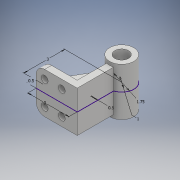
# Autodesk Inventor part: 7d
Saved by Autodesk Inventor 2018 (Build 220112000, 112)
## iProperties
Created: 2018-10-23
Part Number: 7d
Material: Generic
Document SubType Name: Modeling
Designer: Jerry
Density: 1 g/cm^3
Appearance: Default
Author: Jerry
Autodesk Inventor part; units mm, degrees
ref_plane "YZ Plane" through (0, 0, 0) normal (1, 0, 0) x (0, 1, 0)
ref_plane "XZ Plane" through (0, 0, 0) normal (0, 1, 0) x (-1, 0, 0)
ref_plane "XY Plane" through (0, 0, 0) normal (0, 0, 1) x (1, 0, 0)
sketch "Sketch1" plane through (0, 0, 0) normal (0, 0, 1) x (1, 0, 0)
  line L0 (0, 0) -> (0, 0.5)
  line L1 (0, 0.5) -> (2.5, 0.5)
  line L2 (2.5, 0.5) -> (2.5, 2.6615)
  line L3 (0, 0) -> (3, 0)
  line L4 (3, 0) -> (3, 2.6615)
  circle A0 centre (2.75, 3.5) radius 0.5
  circle A1 centre (2.75, 3.5) radius 0.875
  line L5 (0, 0.5) -> (1.993, 3.9388)
  dimension "d0" = 0.5
  dimension "d1" = 0.5
  dimension "d2" = 3
  dimension "d3" = 1
  dimension "d4" = 1.75
  dimension "d20" = 3
  constraints: 12 end point, 3 perpendicular, 3 point on circle, 2 centre point, 1 coincident, 1 horizontal, 1 horizontal alignment, 1 tangent, 1 vertical
  measures "d0" distance between parallel lines of L3 L1
  measures "d1" distance between parallel lines of L4 L2
  measures "d2" distance from line of L1 A0.centre
  measures "d3" diameter of A0
  measures "d4" diameter of A1
  measures "d20" distance from line of L0.start L4
sketch "Sketch2" plane through (0, 0, 0) normal (0, 1, 0) x (-1, 0, 0)
  line L0 (0.7553, 0) -> (-3.6259, 0) projected
  line L1 (0, 0) -> (0, -0.875)
  arc A0 (-0.625, -1.5) -> (0, -0.875) centre (-0.625, -0.875) ccw
  line L2 (-0.625, -1.5) -> (-3, -1.5)
  line L3 (-3, -1.5) -> (-3, 1.5)
  line L4 (-3, 1.5) -> (-0.625, 1.5)
  arc A1 (0, 0.875) -> (-0.625, 1.5) centre (-0.625, 0.875) ccw
  line L5 (0, 0.875) -> (0, 0)
  line L6 (0, -0.25) -> (-2.5, -0.25)
  line L7 (-2.5, -0.25) -> (-2.5, -1.5)
  line L8 (0, 0.25) -> (-2.5, 0.25)
  line L9 (-2.5, 0.25) -> (-2.5, 1.5)
  circle A2 centre (-0.625, -0.875) radius 0.25
  circle A3 centre (-1.875, -0.875) radius 0.25
  circle A4 centre (-0.625, 0.875) radius 0.25
  circle A5 centre (-1.875, 0.875) radius 0.25
  point P0 (-0.625, -0.875)
  point P1 (-1.875, -0.875)
  point P2 (-1.875, 0.875)
  point P3 (-0.625, 0.875)
  dimension "d5" = 1.75
  dimension "d6" = 1.25
  dimension "d7" = 0.625
  dimension "d8" = 1.25
  dimension "d9" = 2.5
  dimension "d10" = 3
  dimension "d11" = 0.5
  dimension "d14" = 1.25
  dimension "d17" = 1.75
  dimension "d21" = 3
  constraints: 18 end point, 7 perpendicular, 7 point on line, 6 centre point, 4 point on circle, 4 tangent, 2 coincident, 2 horizontal alignment, 2 vertical, 2 vertical alignment, 1 horizontal, 1 parallel, 1 symmetric about line, 10 other
  measures "d5" distance of point (-0.625, 0.875) point (-0.625, -0.875)
  measures "d6" distance of point (-1.875, -0.875) point (-0.625, -0.875)
  measures "d7" radius of A0
  measures "d8" distance between parallel lines of L2 L6
  measures "d9" distance of L6.start L6.end
  measures "d10" distance between parallel lines of L1 L3
  measures "d11" diameter of A2
  measures "d14" distance of A2.centre A3.centre
  measures "d17" distance of A2.centre A4.centre
  measures "d21" distance of L2.end L3.end
extrude "Extrusion1" add sketch "Sketch1" along normal mid plane 3 contours L0 L1 L2 A1 L4 L3
extrude "Extrusion2" add sketch "Sketch1" along normal mid plane 3.5 contours A1
extrude "Extrusion3" add sketch "Sketch1" along normal mid plane 0.5 contours L5 A1 L2 L1
fillet "Fillet1" radius 0.625 2 edges at (0, 0.25, 1.5) (0, 0.25, -1.5)
extrude "Extrusion4" cut sketch "Sketch2" along normal blind 0.6 contours A2 | A3 | A4 | A5
fillet "Fillet2" radius 0.05 2 edges at (2.5, 1.5807, -0.25) (2.5, 1.5807, 0.25)
body "Solid1"
